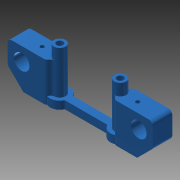
# Autodesk Inventor part: spacer stepperM n rail
Saved by Autodesk Inventor 2013 SP2 (Build 170200200, 200)
## iProperties
Created: 2017-02-21
Part Number: spacer stepperM n rail
Material: Generic
Document SubType Name: Modeling
Designer: Herman de Vries
Density: 1 g/cm^3
Mass: 7.01236 g
Surface Area: 44.8839 cm^2
Volume: 7.01236 cm^3
Author: Herman de Vries
Autodesk Inventor part; units mm, degrees
note: some values were not read from the file. Chosen so that the rebuilt part matches the saved one: sketch regions of "Extrusion2".
ref_plane "YZ Plane" through (0, 0, 0) normal (1, 0, 0) x (0, 1, 0)
ref_plane "XZ Plane" through (0, 0, 0) normal (0, 1, 0) x (-1, 0, 0)
ref_plane "XY Plane" through (0, 0, 0) normal (0, 0, 1) x (1, 0, 0)
sketch "Sketch1" plane through (0, 0, 0) normal (0, 0, 1) x (1, 0, 0)
  circle A0 centre (0, 0) radius 1.65
  circle A1 centre (0, 0) radius 3
  circle A2 centre (31, 0) radius 1.65
  circle A3 centre (31, 0) radius 3
  dimension "d0" = 3.3
  dimension "d1" = 6
  dimension "d22" = 31
  constraints: 4 centre point, 3 coincident, 2 equal radius
  measures "d0" diameter of A0
  measures "d1" diameter of A1
  measures "d22" distance of A2.centre point (0, 0)
extrude "Extrusion1" add sketch "Sketch1" along normal blind 26
sketch "Sketch2" plane through (0, 0, 0) normal (0, 0, -1) x (-1, 0, 0)
  circle A0 centre (0, 0) radius 3 projected
  circle A1 centre (0, 0) radius 5
  circle A2 centre (-31, 0) radius 1.65 projected
  circle A3 centre (-31, 0) radius 5
  circle A4 centre (0, 0) radius 1.65 construction
  line L0 (-29.35, 2) -> (-1.65, 2)
  line L1 (-1.65, 2) -> (-1.65, -2)
  line L2 (-1.65, -2) -> (-29.35, -2)
  line L3 (-29.35, -2) -> (-29.35, 2)
  point P0 (-1.65, 0)
  dimension "d4" = 10
  dimension "d7" = 4
  constraints: 8 end point, 2 centre point, 2 coincident, 2 parallel, 2 tangent, 1 equal radius, 1 horizontal, 1 horizontal alignment, 1 midpoint, 1 perpendicular
  measures "d4" diameter of A1
  measures "d7" distance between parallel lines of L2 L0
extrude "Extrusion2" add sketch "Sketch2" against normal blind 4 contours A0 L0 A1 L2 | L0 L1 L2 A0 | A0 L2 A1 L0 | A1 L2 A3 L0 | L0 L3 L2 A3 | A3 L2 L3 L0 picked at (-2.1, 0)
sketch "Sketch3" plane through (0, 0, 0) normal (0, 0, -1) x (-1, 0, 0)
  line L0 (-52.65, -5) -> (-32.65, -5)
  line L1 (-32.65, -5) -> (-32.65, 5)
  line L2 (-32.65, 5) -> (-52.65, 5)
  line L3 (-52.65, 5) -> (-52.65, -5)
  line L4 (1.65, 5) -> (21.65, 5)
  line L5 (21.65, 5) -> (21.65, -5)
  line L6 (21.65, -5) -> (1.65, -5)
  line L7 (1.65, -5) -> (1.65, 5)
  circle A0 centre (0, 0) radius 1.65 construction
  circle A1 centre (-31, 0) radius 1.65 construction
  arc A2 (-26.4174, 2) -> (-26.4174, -2) centre (-31, 0) ccw construction
  arc A3 (-4.5826, -2) -> (-4.5826, 2) centre (0, 0) ccw construction
  point P0 (-32.65, 0)
  point P1 (1.65, 0)
  dimension "d8" = 20
  dimension "d10" = 20
  constraints: 16 end point, 4 parallel, 4 tangent, 2 horizontal, 2 horizontal alignment, 2 midpoint, 2 perpendicular
  measures "d8" distance of L1.end L2.end
  measures "d10" distance of L4.start L4.end
extrude "Extrusion3" add sketch "Sketch3" against normal blind 20
sketch "Sketch4" plane through (32.65, 5, 0) normal (0, 1, 0) x (1, 0, 0)
  circle A0 centre (-47.15, -13) radius 4
  circle A1 centre (12.85, -13) radius 4
  line L0 (-34.3, -20) -> (-54.3, -20) projected
  line L1 (20, -20) -> (0, -20) projected
  line L2 (-34.3, 0) -> (-54.3, 0) projected
  line L3 (20, 0) -> (20, -20) projected
  line L4 (-54.3, 0) -> (-54.3, -20) projected
  point P0 (-32.65, 0)
  point P1 (-44.3, -20)
  point P2 (10, -20)
  dimension "d13" = 8
  dimension "d14" = 8
  dimension "d15" = 13
  dimension "d23" = 60
  dimension "d24" = 7.15
  dimension "d25" = 7.15
  constraints: 2 centre point, 2 midpoint, 1 horizontal alignment
  measures "d13" diameter of A0
  measures "d14" diameter of A1
  measures "d15" distance from line of A0.centre L2
  measures "d23" distance of A1.centre A0.centre
  measures "d24" distance from line of L3 A1.centre
  measures "d25" distance from line of A0.centre L4
extrude "Extrusion4" cut sketch "Sketch4" against normal blind 20
chamfer "Chamfer1" distance 8 angle 45 2 edges at (52.65, 0, 0) (-21.65, 0, 0)
fillet "Fillet1" radius 2 12 edges at (32.65, 2.5055, 12) (32.65, -2.5055, 12) (32.65, 5, 10) (-1.65, 2.5055, 12) (-1.65, -2.5055, 12) (-1.65, 5, 10) (-1.65, -5, 10) (32.65, -5, 10) (52.65, 0, 20) (52.65, 0, 8) (-21.65, 0, 8) (-21.65, 0, 20)
sketch "Sketch5" plane through (0, 0, 20) normal (0, 0, 1) x (1, 0, 0)
  line L0 (-19.65, -5) -> (-19.65, 5) projected
  arc A0 (0.21, 2.9926) -> (0.21, -2.9926) centre (0, 0) ccw projected
  circle A1 centre (-9, 0) radius 1
  circle A2 centre (40, 0) radius 1
  arc A3 (30.79, -2.9926) -> (30.79, 2.9926) centre (31, 0) ccw projected
  point P0 (-19.65, 0)
  dimension "d26" = 2
  dimension "d27" = 2
  dimension "d28" = 5
  dimension "d29" = 5
  constraints: 2 centre point, 2 horizontal alignment, 1 midpoint
  measures "d26" diameter of A1
  measures "d27" diameter of A2
extrude "Extrusion5" cut sketch "Sketch5" against normal blind 10
equation "\"d10\" = d8"
equation "\"d24\" = d25"
equation "\"d29\" = d28"
body "Solid1"
